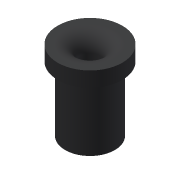
# Autodesk Inventor part: Bushing Drill
Saved by Autodesk Inventor 2022 Beta2 (Build 260130000, 130) ContinuousBuild 0
## iProperties
Created: 2006-01-31
Part Number: Bushing Drill
Document SubType Name: Modeling
Designer: landrews
Stock Number: Bushing Drill
Density: 1 g/cm^3
Material: Generic
Appearance: Generic
Author: landrews
Autodesk Inventor part; units mm, degrees
ref_plane "YZ Plane" through (0, 0, 0) normal (1, 0, 0) x (0, 1, 0)
ref_plane "XZ Plane" through (0, 0, 0) normal (0, 1, 0) x (-1, 0, 0)
ref_plane "XY Plane" through (0, 0, 0) normal (0, 0, 1) x (1, 0, 0)
sketch "Sketch1" plane through (0, 0, 0) normal (0, 0, 1) x (1, 0, 0)
  line L0 (-6, 0) -> (8, 0) projected
  line L1 (0, 8) -> (0, -6) projected
  circle A0 centre (0, 0) radius 5
  dimension "d0" = 10
  constraints: 2 point on line, 1 centre point
  measures "d0" diameter of A0
extrude "Extrusion1" add sketch "Sketch1" along normal blind 13
sketch "Sketch2" plane through (0, 0, 13) normal (0, 0, 1) x (1, 0, 0)
  circle A0 centre (0, 0) radius 5 construction
  circle A1 centre (0, 0) radius 6.5
  dimension "d3" = 13
  constraints: 1 centre point, 1 coincident
  measures "d3" diameter of A1
extrude "Extrusion2" add sketch "Sketch2" along normal blind 3
hole "Hole1" at (0, 0, 16) direction (0, 0, -1) diameter 4 end through all
fillet "Fillet1" radius 3 1 edges at (0, 2, 16)
fillet "Fillet2" radius 2 1 edges at (0, 2, 0)
body "Solid1"
